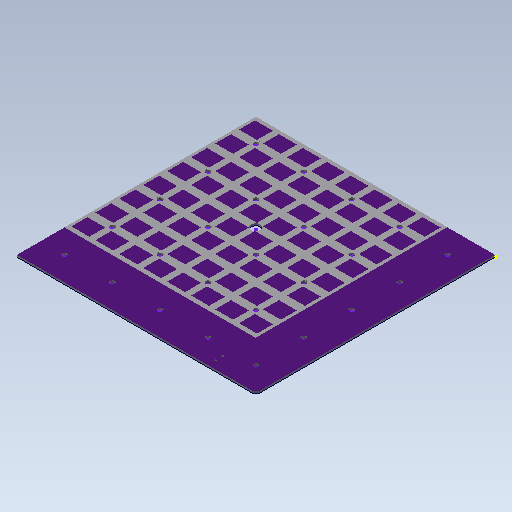
# Autodesk Inventor part: J010131A
Saved by Autodesk Inventor 2020.3 (Build 243373000, 373)
## iProperties
RuleStatus: InUse
AfterDocSave0: file://Part Number Cleaner
Created: 2022-03-30
Part Number: J010131A
Material: Generic
Catalog Web Link: https://www.janelia.org/
Vendor: HHMI: JRC - jET
Document SubType Name: Modeling
Designer: goulett
Density: 1 g/cm^3
Appearance: Default
Description: 5X5 LED BOARD RGR + IR
LAB/DEPT: A. LEE (LAB)
DESIGN DEPARTMENT: HHMI: JRC - jET
ALTERED ITEM PART NUMBER: N/A
ALTERED ITEM VENDOR: N/A
ALTERED ITEM DESCRIPTION: N/A
Title: Standard
Author: goulett
Revision Number: 0
Autodesk Inventor part; units mm, degrees
ref_plane "YZ Plane" through (0, 0, 0) normal (1, 0, 0) x (0, 1, 0)
ref_plane "XZ Plane" through (0, 0, 0) normal (0, 1, 0) x (-1, 0, 0)
ref_plane "XY Plane" through (0, 0, 0) normal (0, 0, 1) x (1, 0, 0)
sketch "Sketch1" plane through (0, 0, 0) normal (0, 1, 0) x (-1, 0, 0)
  line L0 (0, 149.86) -> (0, 0)
  line L1 (0, 149.86) -> (2.286, 152.146)
  line L2 (2.286, 152.146) -> (152.146, 152.146)
  line L3 (152.146, 0) -> (0, 0)
  line L4 (152.146, 0) -> (152.146, 152.146)
  circle A0 centre (91.44, 60.96) radius 2.9972
  circle A1 centre (15.24, 136.906) radius 1.5875
  circle A2 centre (30.861, 147.146) radius 0.8
  circle A3 centre (30.861, 142.646) radius 0.9
  line L5 (30.48, 121.92) -> (152.146, 121.92)
  line L6 (152.146, 121.92) -> (152.146, 0)
  line L7 (152.146, 0) -> (30.48, 0)
  line L8 (30.48, 0) -> (30.48, 121.92)
  circle A4 centre (15.24, 136.906) radius 1.5875
  circle A5 centre (45.72, 136.906) radius 1.5875
  circle A6 centre (76.2, 136.906) radius 1.5875
  circle A7 centre (106.68, 136.906) radius 1.5875
  circle A8 centre (137.16, 136.906) radius 1.5875
  circle A9 centre (137.16, 106.426) radius 1.5875
  circle A10 centre (106.68, 106.426) radius 1.5875
  circle A11 centre (76.2, 106.426) radius 1.5875
  circle A12 centre (45.72, 106.426) radius 1.5875
  circle A13 centre (15.24, 106.426) radius 1.5875
  circle A14 centre (15.24, 75.946) radius 1.5875
  circle A15 centre (137.16, 45.466) radius 1.5875
  circle A16 centre (106.68, 45.466) radius 1.5875
  circle A17 centre (76.2, 45.466) radius 1.5875
  circle A18 centre (45.72, 45.466) radius 1.5875
  circle A19 centre (15.24, 45.466) radius 1.5875
  circle A20 centre (15.24, 14.986) radius 1.5875
  circle A21 centre (45.72, 14.986) radius 1.5875
  circle A22 centre (76.2, 14.986) radius 1.5875
  circle A23 centre (106.68, 14.986) radius 1.5875
  circle A24 centre (137.16, 14.986) radius 1.5875
  circle A25 centre (76.2, 75.946) radius 1.5875
  circle A26 centre (106.68, 75.946) radius 1.5875
  line L9 (35.461, 151.946) -> (35.461, 152.146)
  line L10 (35.461, 152.146) -> (26.361, 152.146)
  line L11 (26.361, 152.146) -> (26.361, 151.846)
  circle A27 centre (137.16, 75.946) radius 1.5875
  circle A28 centre (45.72, 75.946) radius 1.5875
  constraints: 29 centre point, 24 end point
extrude "Extrusion1" add sketch "Sketch1" along normal blind 1.27
sketch "Sketch2" plane through (0, 1.27, 0) normal (0, 1, 0) x (1, 0, 0)
  line L0 (-30.48, 0) -> (-30.48, -121.92) projected
  line L1 (-30.48, -121.92) -> (-152.146, -121.92) projected
  line L2 (0, -149.86) -> (0, 0) projected
  line L3 (-152.146, -152.146) -> (-2.286, -152.146) projected
  line L4 (-152.146, 0) -> (-152.146, -152.146) projected
  line L5 (0, 0) -> (-152.146, 0) projected
  line L6 (0, -149.86) -> (0, 0) projected
  line L7 (-2.286, -152.146) -> (0, -149.86) projected
  line L8 (-152.146, -152.146) -> (-2.286, -152.146) projected
  circle A0 centre (-15.24, -45.466) radius 1.5875 projected
  circle A1 centre (-15.24, -106.426) radius 1.5875 projected
  circle A2 centre (-15.24, -136.906) radius 1.5875 projected
  circle A3 centre (-30.861, -147.146) radius 0.8 projected
  circle A4 centre (-30.861, -142.646) radius 0.9 projected
  circle A5 centre (-45.72, -136.906) radius 1.5875 projected
  circle A6 centre (-76.2, -136.906) radius 1.5875 projected
  circle A7 centre (-106.68, -136.906) radius 1.5875 projected
  circle A8 centre (-137.16, -136.906) radius 1.5875 projected
  circle A9 centre (-15.24, -75.946) radius 1.5875 projected
  circle A10 centre (-15.24, -14.986) radius 1.5875 projected
  circle A11 centre (-137.16, -75.946) radius 1.5875 projected
  circle A12 centre (-76.2, -75.946) radius 1.5875 projected
  circle A13 centre (-106.68, -14.986) radius 1.5875 projected
  circle A14 centre (-45.72, -14.986) radius 1.5875 projected
  circle A15 centre (-76.2, -45.466) radius 1.5875 projected
  circle A16 centre (-106.68, -45.466) radius 1.5875 projected
  circle A17 centre (-137.16, -45.466) radius 1.5875 projected
  circle A18 centre (-45.72, -106.426) radius 1.5875 projected
  circle A19 centre (-76.2, -106.426) radius 1.5875 projected
  circle A20 centre (-106.68, -106.426) radius 1.5875 projected
  circle A21 centre (-137.16, -106.426) radius 1.5875 projected
  circle A22 centre (-91.44, -60.96) radius 2.9972 projected
  circle A23 centre (-45.72, -45.466) radius 1.5875 projected
  circle A24 centre (-76.2, -14.986) radius 1.5875 projected
  circle A25 centre (-137.16, -14.986) radius 1.5875 projected
  circle A26 centre (-106.68, -75.946) radius 1.5875 projected
  circle A27 centre (-45.72, -75.946) radius 1.5875 projected
  line L9 (-150.495, -12.446) -> (-139.065, -12.446)
  line L10 (-139.065, -12.446) -> (-139.065, -2.286)
  line L11 (-139.065, -2.286) -> (-150.495, -2.286)
  line L12 (-150.495, -2.286) -> (-150.495, -12.446)
  line L13 (-152.146, -121.92) -> (-146.4837, -121.92)
  line L14 (-146.4837, -121.92) -> (-146.4837, -118.6688)
  line L15 (-146.4837, -118.6688) -> (-152.146, -118.6688)
  line L16 (-152.146, -118.6688) -> (-152.146, -121.92)
  circle A28 centre (-137.16, -14.986) radius 1.905
  circle A29 centre (-45.72, -14.986) radius 1.905
  circle A30 centre (-137.16, -106.426) radius 1.905
  circle A31 centre (-137.16, -14.986) radius 2.54
  circle A32 centre (-137.16, -14.986) radius 1.5875 projected
  circle A33 centre (-106.68, -14.986) radius 1.905
  circle A34 centre (-76.2, -14.986) radius 1.905
  circle A35 centre (-45.72, -14.986) radius 1.905
  circle A36 centre (-137.16, -45.466) radius 1.905
  circle A37 centre (-106.68, -45.466) radius 1.905
  circle A38 centre (-76.2, -45.466) radius 1.905
  circle A39 centre (-45.72, -45.466) radius 1.905
  circle A40 centre (-137.16, -75.946) radius 1.905
  circle A41 centre (-106.68, -75.946) radius 1.905
  circle A42 centre (-76.2, -75.946) radius 1.905
  circle A43 centre (-45.72, -75.946) radius 1.905
  circle A44 centre (-137.16, -106.426) radius 1.905
  circle A45 centre (-106.68, -106.426) radius 1.905
  circle A46 centre (-76.2, -106.426) radius 1.905
  circle A47 centre (-45.72, -106.426) radius 1.905
  line L17 (-135.255, -2.286) -> (-123.825, -2.286)
  line L18 (-123.825, -2.286) -> (-123.825, -12.446)
  line L19 (-123.825, -12.446) -> (-135.255, -12.446)
  line L20 (-135.255, -12.446) -> (-135.255, -2.286)
  line L21 (-108.585, -12.446) -> (-120.015, -12.446)
  line L22 (-120.015, -12.446) -> (-120.015, -2.286)
  line L23 (-120.015, -2.286) -> (-108.585, -2.286)
  line L24 (-108.585, -2.286) -> (-108.585, -12.446)
  line L25 (-150.495, -27.686) -> (-139.065, -27.686)
  line L26 (-139.065, -27.686) -> (-139.065, -17.526)
  line L27 (-139.065, -17.526) -> (-150.495, -17.526)
  line L28 (-150.495, -17.526) -> (-150.495, -27.686)
  line L29 (-150.495, -42.926) -> (-139.065, -42.926)
  line L30 (-139.065, -42.926) -> (-139.065, -32.766)
  line L31 (-139.065, -32.766) -> (-150.495, -32.766)
  line L32 (-150.495, -32.766) -> (-150.495, -42.926)
  line L33 (-150.495, -58.166) -> (-139.065, -58.166)
  line L34 (-139.065, -58.166) -> (-139.065, -48.006)
  line L35 (-139.065, -48.006) -> (-150.495, -48.006)
  line L36 (-150.495, -48.006) -> (-150.495, -58.166)
  line L37 (-150.495, -73.406) -> (-139.065, -73.406)
  line L38 (-139.065, -73.406) -> (-139.065, -63.246)
  line L39 (-139.065, -63.246) -> (-150.495, -63.246)
  line L40 (-150.495, -63.246) -> (-150.495, -73.406)
  line L41 (-150.495, -88.646) -> (-139.065, -88.646)
  line L42 (-139.065, -88.646) -> (-139.065, -78.486)
  line L43 (-139.065, -78.486) -> (-150.495, -78.486)
  line L44 (-150.495, -78.486) -> (-150.495, -88.646)
  line L45 (-150.495, -103.886) -> (-139.065, -103.886)
  line L46 (-139.065, -103.886) -> (-139.065, -93.726)
  line L47 (-139.065, -93.726) -> (-150.495, -93.726)
  line L48 (-150.495, -93.726) -> (-150.495, -103.886)
  line L49 (-150.495, -119.126) -> (-139.065, -119.126)
  line L50 (-139.065, -119.126) -> (-139.065, -108.966)
  line L51 (-139.065, -108.966) -> (-150.495, -108.966)
  line L52 (-150.495, -108.966) -> (-150.495, -119.126)
  line L53 (-135.255, -12.446) -> (-123.825, -12.446)
  line L54 (-123.825, -12.446) -> (-123.825, -2.286)
  line L55 (-123.825, -2.286) -> (-135.255, -2.286)
  line L56 (-135.255, -2.286) -> (-135.255, -12.446)
  line L57 (-135.255, -27.686) -> (-123.825, -27.686)
  line L58 (-123.825, -27.686) -> (-123.825, -17.526)
  line L59 (-123.825, -17.526) -> (-135.255, -17.526)
  line L60 (-135.255, -17.526) -> (-135.255, -27.686)
  line L61 (-135.255, -42.926) -> (-123.825, -42.926)
  line L62 (-123.825, -42.926) -> (-123.825, -32.766)
  line L63 (-123.825, -32.766) -> (-135.255, -32.766)
  line L64 (-135.255, -32.766) -> (-135.255, -42.926)
  line L65 (-135.255, -58.166) -> (-123.825, -58.166)
  line L66 (-123.825, -58.166) -> (-123.825, -48.006)
  line L67 (-123.825, -48.006) -> (-135.255, -48.006)
  line L68 (-135.255, -48.006) -> (-135.255, -58.166)
  line L69 (-135.255, -73.406) -> (-123.825, -73.406)
  line L70 (-123.825, -73.406) -> (-123.825, -63.246)
  line L71 (-123.825, -63.246) -> (-135.255, -63.246)
  line L72 (-135.255, -63.246) -> (-135.255, -73.406)
  line L73 (-135.255, -88.646) -> (-123.825, -88.646)
  line L74 (-123.825, -88.646) -> (-123.825, -78.486)
  line L75 (-123.825, -78.486) -> (-135.255, -78.486)
  line L76 (-135.255, -78.486) -> (-135.255, -88.646)
  line L77 (-135.255, -103.886) -> (-123.825, -103.886)
  line L78 (-123.825, -103.886) -> (-123.825, -93.726)
  line L79 (-123.825, -93.726) -> (-135.255, -93.726)
  line L80 (-135.255, -93.726) -> (-135.255, -103.886)
  line L81 (-135.255, -119.126) -> (-123.825, -119.126)
  line L82 (-123.825, -119.126) -> (-123.825, -108.966)
  line L83 (-123.825, -108.966) -> (-135.255, -108.966)
  line L84 (-135.255, -108.966) -> (-135.255, -119.126)
  line L85 (-120.015, -12.446) -> (-108.585, -12.446)
  line L86 (-108.585, -12.446) -> (-108.585, -2.286)
  line L87 (-108.585, -2.286) -> (-120.015, -2.286)
  line L88 (-120.015, -2.286) -> (-120.015, -12.446)
  line L89 (-120.015, -27.686) -> (-108.585, -27.686)
  line L90 (-108.585, -27.686) -> (-108.585, -17.526)
  line L91 (-108.585, -17.526) -> (-120.015, -17.526)
  line L92 (-120.015, -17.526) -> (-120.015, -27.686)
  line L93 (-120.015, -42.926) -> (-108.585, -42.926)
  line L94 (-108.585, -42.926) -> (-108.585, -32.766)
  line L95 (-108.585, -32.766) -> (-120.015, -32.766)
  line L96 (-120.015, -32.766) -> (-120.015, -42.926)
  line L97 (-120.015, -58.166) -> (-108.585, -58.166)
  line L98 (-108.585, -58.166) -> (-108.585, -48.006)
  line L99 (-108.585, -48.006) -> (-120.015, -48.006)
  line L100 (-120.015, -48.006) -> (-120.015, -58.166)
  line L101 (-120.015, -73.406) -> (-108.585, -73.406)
  line L102 (-108.585, -73.406) -> (-108.585, -63.246)
  line L103 (-108.585, -63.246) -> (-120.015, -63.246)
  line L104 (-120.015, -63.246) -> (-120.015, -73.406)
  line L105 (-120.015, -88.646) -> (-108.585, -88.646)
  line L106 (-108.585, -88.646) -> (-108.585, -78.486)
  line L107 (-108.585, -78.486) -> (-120.015, -78.486)
  line L108 (-120.015, -78.486) -> (-120.015, -88.646)
  line L109 (-120.015, -103.886) -> (-108.585, -103.886)
  line L110 (-108.585, -103.886) -> (-108.585, -93.726)
  line L111 (-108.585, -93.726) -> (-120.015, -93.726)
  line L112 (-120.015, -93.726) -> (-120.015, -103.886)
  line L113 (-120.015, -119.126) -> (-108.585, -119.126)
  line L114 (-108.585, -119.126) -> (-108.585, -108.966)
  line L115 (-108.585, -108.966) -> (-120.015, -108.966)
  line L116 (-120.015, -108.966) -> (-120.015, -119.126)
  line L117 (-104.775, -12.446) -> (-93.345, -12.446)
  line L118 (-93.345, -12.446) -> (-93.345, -2.286)
  line L119 (-93.345, -2.286) -> (-104.775, -2.286)
  line L120 (-104.775, -2.286) -> (-104.775, -12.446)
  line L121 (-104.775, -27.686) -> (-93.345, -27.686)
  line L122 (-93.345, -27.686) -> (-93.345, -17.526)
  line L123 (-93.345, -17.526) -> (-104.775, -17.526)
  line L124 (-104.775, -17.526) -> (-104.775, -27.686)
  line L125 (-104.775, -42.926) -> (-93.345, -42.926)
  line L126 (-93.345, -42.926) -> (-93.345, -32.766)
  line L127 (-93.345, -32.766) -> (-104.775, -32.766)
  line L128 (-104.775, -32.766) -> (-104.775, -42.926)
  line L129 (-104.775, -58.166) -> (-93.345, -58.166)
  line L130 (-93.345, -58.166) -> (-93.345, -48.006)
  line L131 (-93.345, -48.006) -> (-104.775, -48.006)
  line L132 (-104.775, -48.006) -> (-104.775, -58.166)
  line L133 (-104.775, -73.406) -> (-93.345, -73.406)
  line L134 (-93.345, -73.406) -> (-93.345, -63.246)
  line L135 (-93.345, -63.246) -> (-104.775, -63.246)
  line L136 (-104.775, -63.246) -> (-104.775, -73.406)
  line L137 (-104.775, -88.646) -> (-93.345, -88.646)
  line L138 (-93.345, -88.646) -> (-93.345, -78.486)
  line L139 (-93.345, -78.486) -> (-104.775, -78.486)
  line L140 (-104.775, -78.486) -> (-104.775, -88.646)
  line L141 (-104.775, -103.886) -> (-93.345, -103.886)
  line L142 (-93.345, -103.886) -> (-93.345, -93.726)
  line L143 (-93.345, -93.726) -> (-104.775, -93.726)
  line L144 (-104.775, -93.726) -> (-104.775, -103.886)
  line L145 (-104.775, -119.126) -> (-93.345, -119.126)
  line L146 (-93.345, -119.126) -> (-93.345, -108.966)
  line L147 (-93.345, -108.966) -> (-104.775, -108.966)
  line L148 (-104.775, -108.966) -> (-104.775, -119.126)
  line L149 (-89.535, -12.446) -> (-78.105, -12.446)
  line L150 (-78.105, -12.446) -> (-78.105, -2.286)
  line L151 (-78.105, -2.286) -> (-89.535, -2.286)
  line L152 (-89.535, -2.286) -> (-89.535, -12.446)
  line L153 (-89.535, -27.686) -> (-78.105, -27.686)
  line L154 (-78.105, -27.686) -> (-78.105, -17.526)
  line L155 (-78.105, -17.526) -> (-89.535, -17.526)
  line L156 (-89.535, -17.526) -> (-89.535, -27.686)
  line L157 (-89.535, -42.926) -> (-78.105, -42.926)
  line L158 (-78.105, -42.926) -> (-78.105, -32.766)
  line L159 (-78.105, -32.766) -> (-89.535, -32.766)
  line L160 (-89.535, -32.766) -> (-89.535, -42.926)
  line L161 (-89.535, -58.166) -> (-78.105, -58.166)
  line L162 (-78.105, -58.166) -> (-78.105, -48.006)
  line L163 (-78.105, -48.006) -> (-89.535, -48.006)
  line L164 (-89.535, -48.006) -> (-89.535, -58.166)
  line L165 (-89.535, -73.406) -> (-78.105, -73.406)
  line L166 (-78.105, -73.406) -> (-78.105, -63.246)
  line L167 (-78.105, -63.246) -> (-89.535, -63.246)
  line L168 (-89.535, -63.246) -> (-89.535, -73.406)
  line L169 (-89.535, -88.646) -> (-78.105, -88.646)
  line L170 (-78.105, -88.646) -> (-78.105, -78.486)
  line L171 (-78.105, -78.486) -> (-89.535, -78.486)
  line L172 (-89.535, -78.486) -> (-89.535, -88.646)
  line L173 (-89.535, -103.886) -> (-78.105, -103.886)
  line L174 (-78.105, -103.886) -> (-78.105, -93.726)
  line L175 (-78.105, -93.726) -> (-89.535, -93.726)
  line L176 (-89.535, -93.726) -> (-89.535, -103.886)
  line L177 (-89.535, -119.126) -> (-78.105, -119.126)
  line L178 (-78.105, -119.126) -> (-78.105, -108.966)
  line L179 (-78.105, -108.966) -> (-89.535, -108.966)
  line L180 (-89.535, -108.966) -> (-89.535, -119.126)
  line L181 (-74.295, -12.446) -> (-62.865, -12.446)
  line L182 (-62.865, -12.446) -> (-62.865, -2.286)
  line L183 (-62.865, -2.286) -> (-74.295, -2.286)
  line L184 (-74.295, -2.286) -> (-74.295, -12.446)
  line L185 (-74.295, -27.686) -> (-62.865, -27.686)
  line L186 (-62.865, -27.686) -> (-62.865, -17.526)
  line L187 (-62.865, -17.526) -> (-74.295, -17.526)
  line L188 (-74.295, -17.526) -> (-74.295, -27.686)
  line L189 (-74.295, -42.926) -> (-62.865, -42.926)
  line L190 (-62.865, -42.926) -> (-62.865, -32.766)
  line L191 (-62.865, -32.766) -> (-74.295, -32.766)
  line L192 (-74.295, -32.766) -> (-74.295, -42.926)
  line L193 (-74.295, -58.166) -> (-62.865, -58.166)
  line L194 (-62.865, -58.166) -> (-62.865, -48.006)
  line L195 (-62.865, -48.006) -> (-74.295, -48.006)
  line L196 (-74.295, -48.006) -> (-74.295, -58.166)
  line L197 (-74.295, -73.406) -> (-62.865, -73.406)
  line L198 (-62.865, -73.406) -> (-62.865, -63.246)
  line L199 (-62.865, -63.246) -> (-74.295, -63.246)
  line L200 (-74.295, -63.246) -> (-74.295, -73.406)
  line L201 (-74.295, -88.646) -> (-62.865, -88.646)
  line L202 (-62.865, -88.646) -> (-62.865, -78.486)
  line L203 (-62.865, -78.486) -> (-74.295, -78.486)
  line L204 (-74.295, -78.486) -> (-74.295, -88.646)
  line L205 (-74.295, -103.886) -> (-62.865, -103.886)
  line L206 (-62.865, -103.886) -> (-62.865, -93.726)
  line L207 (-62.865, -93.726) -> (-74.295, -93.726)
  line L208 (-74.295, -93.726) -> (-74.295, -103.886)
  line L209 (-74.295, -119.126) -> (-62.865, -119.126)
  line L210 (-62.865, -119.126) -> (-62.865, -108.966)
  line L211 (-62.865, -108.966) -> (-74.295, -108.966)
  line L212 (-74.295, -108.966) -> (-74.295, -119.126)
  line L213 (-59.055, -12.446) -> (-47.625, -12.446)
  line L214 (-47.625, -12.446) -> (-47.625, -2.286)
  line L215 (-47.625, -2.286) -> (-59.055, -2.286)
  line L216 (-59.055, -2.286) -> (-59.055, -12.446)
  line L217 (-59.055, -27.686) -> (-47.625, -27.686)
  line L218 (-47.625, -27.686) -> (-47.625, -17.526)
  line L219 (-47.625, -17.526) -> (-59.055, -17.526)
  line L220 (-59.055, -17.526) -> (-59.055, -27.686)
  line L221 (-59.055, -42.926) -> (-47.625, -42.926)
  line L222 (-47.625, -42.926) -> (-47.625, -32.766)
  line L223 (-47.625, -32.766) -> (-59.055, -32.766)
  line L224 (-59.055, -32.766) -> (-59.055, -42.926)
  line L225 (-59.055, -58.166) -> (-47.625, -58.166)
  line L226 (-47.625, -58.166) -> (-47.625, -48.006)
  line L227 (-47.625, -48.006) -> (-59.055, -48.006)
  line L228 (-59.055, -48.006) -> (-59.055, -58.166)
  line L229 (-59.055, -73.406) -> (-47.625, -73.406)
  line L230 (-47.625, -73.406) -> (-47.625, -63.246)
  line L231 (-47.625, -63.246) -> (-59.055, -63.246)
  line L232 (-59.055, -63.246) -> (-59.055, -73.406)
  line L233 (-59.055, -88.646) -> (-47.625, -88.646)
  line L234 (-47.625, -88.646) -> (-47.625, -78.486)
  line L235 (-47.625, -78.486) -> (-59.055, -78.486)
  line L236 (-59.055, -78.486) -> (-59.055, -88.646)
  line L237 (-59.055, -103.886) -> (-47.625, -103.886)
  line L238 (-47.625, -103.886) -> (-47.625, -93.726)
  line L239 (-47.625, -93.726) -> (-59.055, -93.726)
  line L240 (-59.055, -93.726) -> (-59.055, -103.886)
  line L241 (-59.055, -119.126) -> (-47.625, -119.126)
  line L242 (-47.625, -119.126) -> (-47.625, -108.966)
  line L243 (-47.625, -108.966) -> (-59.055, -108.966)
  line L244 (-59.055, -108.966) -> (-59.055, -119.126)
  line L245 (-43.815, -12.446) -> (-32.385, -12.446)
  line L246 (-32.385, -12.446) -> (-32.385, -2.286)
  line L247 (-32.385, -2.286) -> (-43.815, -2.286)
  line L248 (-43.815, -2.286) -> (-43.815, -12.446)
  line L249 (-43.815, -27.686) -> (-32.385, -27.686)
  line L250 (-32.385, -27.686) -> (-32.385, -17.526)
  line L251 (-32.385, -17.526) -> (-43.815, -17.526)
  line L252 (-43.815, -17.526) -> (-43.815, -27.686)
  line L253 (-43.815, -42.926) -> (-32.385, -42.926)
  line L254 (-32.385, -42.926) -> (-32.385, -32.766)
  line L255 (-32.385, -32.766) -> (-43.815, -32.766)
  line L256 (-43.815, -32.766) -> (-43.815, -42.926)
  line L257 (-43.815, -58.166) -> (-32.385, -58.166)
  line L258 (-32.385, -58.166) -> (-32.385, -48.006)
  line L259 (-32.385, -48.006) -> (-43.815, -48.006)
  line L260 (-43.815, -48.006) -> (-43.815, -58.166)
  line L261 (-43.815, -73.406) -> (-32.385, -73.406)
  line L262 (-32.385, -73.406) -> (-32.385, -63.246)
  line L263 (-32.385, -63.246) -> (-43.815, -63.246)
  line L264 (-43.815, -63.246) -> (-43.815, -73.406)
  line L265 (-43.815, -88.646) -> (-32.385, -88.646)
  line L266 (-32.385, -88.646) -> (-32.385, -78.486)
  line L267 (-32.385, -78.486) -> (-43.815, -78.486)
  line L268 (-43.815, -78.486) -> (-43.815, -88.646)
  line L269 (-43.815, -103.886) -> (-32.385, -103.886)
  line L270 (-32.385, -103.886) -> (-32.385, -93.726)
  line L271 (-32.385, -93.726) -> (-43.815, -93.726)
  line L272 (-43.815, -93.726) -> (-43.815, -103.886)
  line L273 (-43.815, -119.126) -> (-32.385, -119.126)
  line L274 (-32.385, -119.126) -> (-32.385, -108.966)
  line L275 (-32.385, -108.966) -> (-43.815, -108.966)
  line L276 (-43.815, -108.966) -> (-43.815, -119.126)
  point P0 (-2.286, -152.146)
  point P1 (-93.3784, -63.246)
  point P2 (-89.5016, -63.246)
  point P3 (-89.535, -63.2739)
  point P4 (-93.345, -63.2739)
  dimension "d4" = 11.43
  dimension "d5" = 10.16
  dimension "d9" = 3.2512
  dimension "d10" = 3.81
  dimension "d11" = 3.81
  dimension "d12" = 3.81
  dimension "d13" = 5.08
  dimension "d16" = 30.48
  dimension "d19" = 30.48
  dimension "d22" = 11.43
  dimension "d23" = 11.43
  dimension "d24" = 10.16
  dimension "d27" = 15.24
  dimension "d30" = 15.24
  constraints: 536 end point, 19 centre point, 8 parallel, 6 horizontal, 4 perpendicular, 4 tangent, 3 coincident, 3 collinear, 2 vertical, 1 concentric, 534 other
  measures "d4" distance of L11.end L10.end
  measures "d5" distance of L10.end L9.end
  measures "d9" distance of L14.end L13.end
  measures "d10" diameter of A28
  measures "d11" diameter of A29
  measures "d12" diameter of A30
  measures "d13" diameter of A31
  measures "d16" distance of A28.centre A33.centre
  measures "d19" distance of A28.centre A36.centre
  measures "d22" distance of L18.end L19.end
  measures "d23" distance of L22.end L23.end
  measures "d24" distance of L21.end L22.end
  measures "d27" distance of L9.start L25.start
  measures "d30" distance of L9.start L53.start
extrude "Extrusion2" add sketch "Sketch2" along normal blind 0.0254 contours L0 L1 L14 L49 L50 L51 L52 L15 L4 L5 | L1 L4 L15 L52 L49 L14
equation "\"d11\" = d10"
equation "\"d12\" = d10"
body "Solid1"
